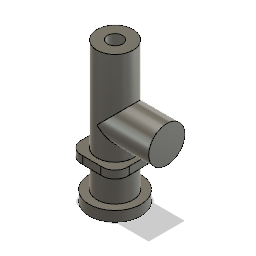
Joint_Assembly v15 (Autodesk Fusion 360 archive; units mm, degrees)
design "Elbow_Joint_Axle"
Autodesk Fusion 360 part; units mm, degrees
cylinder "CylinderPrimitive1" add diameter 14 height 52 placed x (1, 0, 0) y (0, 0, -1) z (0, 1, 0) at (0, 0, 0)
sketch "Sketch2" plane through (0, 52, 0) normal (0, 1, 0) x (-1, 0, 0)
  circle A0 centre (0, 0) radius 7
  circle A1 centre (0, 0) radius 2.9
  dimension "d3" = 5.8
  constraint coincident A0.centre A1.centre
  measures "d3" diameter of A1
extrude "Extrude1" cut sketch "Sketch2" against normal blind 6 contours A1
move_face "MoveFace1" to x (1, 0, 0) y (0, 1, 0) z (0, 0, 1) at (0, 2, 0) 1 faces at (6.9652, 34.6667, 0.697)
sketch "Sketch6" plane through (0, 0, 0) normal (0, -1, 0) x (1, 0, 0)
  circle A0 centre (0, 0) radius 7
  circle A1 centre (0, 0) radius 10
  constraint concentric A0 A1
extrude "Extrude2" add sketch "Sketch6" against normal blind 2
move_body "Move3" bodies 1 to x (1, 0, 0) y (0, 1, 0) z (0, 0, 1) at (0, 2, 0)
extrude "Extrude3" add 1 faces at (3.4521, 2, 1.6624) along direction (0, -1, 0) blind 2
sketch "Sketch9" plane through (0, 0, 0) normal (1, 0, 0) x (0, 0, -1)
  circle A0 centre (0, 29) radius 7
extrude "Extrude5" add sketch "Sketch9" along normal blind 20
sketch "Sketch10" plane through (0, 0, 0) normal (1, 0, 0) x (0, 0, -1)
  line L0 (-7, 17.5) -> (-7, 15)
  line L1 (7, 17.5) -> (7, 15)
  line L2 (-7, 15) -> (-7, 17.5)
  line L3 (-7, 17.5) -> (-7, 18)
  line L4 (-7, 18) -> (7, 18)
  line L5 (7, 18) -> (7, 17.5)
  line L6 (-7, 15) -> (7, 15)
  constraint perpendicular L0 L4
  constraint perpendicular L1 L6
extrude "Extrude9" add sketch "Sketch10" along normal mid plane 18
extrude "Extrude10" add 1 faces at (3, 17, -7) along direction (0, 0, -1) blind 2
extrude "Extrude11" add 1 faces at (6, 17, 7) along direction (0, 0, 1) blind 2
fillet "Fillet2" radius 5.5 curvature continuous 4 edges at (9, 16.5, 9) (9, 16.5, -9) (-9, 16.5, 9) (-9, 16.5, -9)
